2.5mm top thin (Autodesk Fusion 360 design; units mm, degrees)
Autodesk Fusion 360 part; units mm, degrees
note: some values were not read from the file. Chosen so that the rebuilt part matches the saved one: which bodies a step acts on. Set by a fixed rule: which sketch regions a step uses.
sketch "Sketch1" plane through (0, 0, 0) normal (0, 0, 1) x (1, 0, 0)
  line L0 (-28.9023, 0) -> (0, 0) construction
  line L1 (0, 0) -> (0, 16.228) construction
  line L2 (0, 16.228) -> (-28.9023, 16.228) construction
  line L3 (-28.9023, 16.228) -> (-28.9023, 0) construction
  dimension "d1" = 3
  text T0 "2.5 mm top thin" font "Arial" height 3 align right bottom in box 28.9023 x 16.228 at (-28.9023, 0) x (1, 0) y (0, 1) spacing 1
  constraint coincident L0.end
extrude "Extrude1" add sketch "Sketch1" along normal blind 1 text T0 makes body 1 at (-21.2067, 1.1003, 0) makes body 2 at (-23.9754, 2.8417, 0) makes body 3 at (-27.6378, 0.118, 0) makes body 4 at (-5.028, 1, 0.3333) makes body 5 at (-1.766, 0.7244, 0.3333) makes body 6 at (-5.8806, 1.0464, 0) makes body 7 at (-2.6951, 2.7176, 0.3333) makes body 8 at (-12.0182, 1.2368, 0) makes body 9 at (-17.7156, 1.1003, 0) makes body 10 at (-2.6951, 0.7244, 0.3333) makes body 11 at (-25.7449, 0.4195, 0.3333) makes body 12 at (-12.8711, 1.0464, 0) makes body 13 at (-9.6876, 0.1692, 0.3333)
sketch "Sketch2" plane through (0, 0, 0) normal (0, 0, 1) x (1, 0, 0)
  line L0 (-29, 3.8666) -> (1.3214, 3.8666)
  line L1 (1.3214, 3.8666) -> (1.3214, -1.8666)
  line L2 (1.3214, -1.8666) -> (-29, -1.8666)
  line L3 (-29, -1.8666) -> (-29, 3.8666)
  circle A0 centre (1.3214, 1) radius 2.8666
  circle A1 centre (-29, 1) radius 2.8666
  constraint horizontal L0
  constraint vertical L1
  constraint horizontal L2
  constraint vertical L3
  constraint coincident L1.end A0
  constraint tangent L2 A0
  constraint coincident L0.end A0
  constraint coincident L2.end A1
  constraint tangent L2 A1
  constraint coincident L0.start A1
extrude "Extrude2" add sketch "Sketch2" against normal blind 1 bodies 1 2 3
